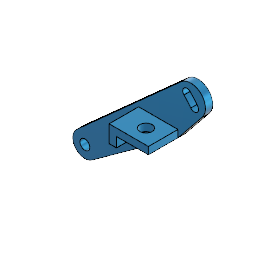
5015 Layer Fan Bracket (Autodesk Fusion 360 design; units mm, degrees)
Autodesk Fusion 360 part; units mm, degrees
ref_plane "WorkPlane1" through (0, 0, 0) normal (0, 0, 1) x (1, 0, 0)
sketch "Sketch1" plane through (0, 0, 0) normal (0, 0, 1) x (1, 0, 0)
  circle A0 centre (-26.3807, -22.7935) radius 5
  circle A1 centre (16.75, 14.4724) radius 6
  circle A2 centre (-26.3807, -22.7935) radius 2
  circle A3 centre (16.75, 14.4724) radius 1.75 construction
  line L0 (0, 0) -> (19.9948, 0) construction
  line L1 (-26.3807, -22.7935) -> (16.75, 14.4724) construction
  line L2 (22.75, 14.4724) -> (30.5, 14.4724) construction
  line L3 (-1.5, 1.4724) -> (-1.5, -1.5276)
  line L4 (11.5, -1.5276) -> (-1.5, -1.5276)
  line L5 (11.5, -1.5276) -> (11.5, 1.4724)
  line L6 (-1.5, 1.4724) -> (11.5, 1.4724)
  arc A4 (-24.5603, -21.835) -> (-27.5407, -24.5029) centre (-26.0505, -23.169) ccw construction
  arc A5 (-28.5639, -23.3119) -> (-25.4917, -20.7503) centre (-27.0278, -22.0311) ccw construction
  line L7 (-29.7155, -19.068) -> (12.7482, 18.9429)
  arc A6 (19.563, 13.7492) -> (16.4427, 17.3605) centre (-4.8153, -4.1606) ccw
  arc A7 (16.7424, 11.677) -> (19.563, 13.7492) centre (18.1527, 12.7131) ccw
  arc A8 (16.7424, 11.677) -> (13.9831, 14.8705) centre (-4.8153, -4.1606) ccw
  arc A9 (16.4427, 17.3605) -> (13.9831, 14.8705) centre (15.2129, 16.1155) ccw
  arc A10 (18.1527, 12.7131) -> (15.2129, 16.1155) centre (-4.8153, -4.1606) ccw construction
  line L8 (-1.5, 1.4724) -> (-6.7689, 1.4724) construction
  line L9 (-1.5, -1.5276) -> (-10.1203, -1.5276) construction
  line L10 (11.5, 1.4724) -> (14.108, 1.4724) construction
  line L11 (21.4103, 10.6932) -> (11.5, -1.5276)
  line L12 (-23.4475, -26.8427) -> (11.5, -1.5276)
  dimension "d5477" = 10
  dimension "d5478" = 12
  dimension "d2" = 4
  dimension "d3" = 3.5
  dimension "d4" = 16.75
  dimension "d5" = 57
  dimension "d6" = 40.828
  dimension "d27" = 2.75
  dimension "d48" = 13
  dimension "d49" = 13
  dimension "d50" = 3
  dimension "d51" = 5.25
  dimension "d54" = 2
  measures "d5477" diameter of A0
  measures "d5478" diameter of A1
  measures "d2" diameter of A2
  measures "d3" diameter of A3
  measures "d4" distance of L0.start
  measures "d5" distance of L0.start
  measures "d6" angle of L0 L1
extrude "Extrude1" add sketch "Sketch1" along normal blind 3 contours A0 | L3 L4 L5 L6 | A0 A1 L7 L11 L12 | A1
extrude "Extrude5" add sketch "Sketch1" along normal blind 15 contours L3 L4 L5 L6
hole "Hole3" at (4.5, 1.4724, 9) direction (0, -1, 0) diameter 5 depth 6 tip angle 118
sketch "Sketch6" plane through (0, 1.4724, 0) normal (0, 1, 0) x (-1, 0, 0)
  circle A0 centre (-4.5, 9) radius 2.5
  line L0 (1.5, 15) -> (-11.5, 15)
  line L1 (-11.5, 15) -> (-11.5, 3)
  line L2 (1.5, 3) -> (1.5, 15)
  line L3 (-11.5, 3) -> (1.5, 3)
  line L4 (-14.5, 18) -> (-14.5, 0)
  line L5 (-14.5, 0) -> (4.5, 0)
  line L6 (4.5, 0) -> (4.5, 18)
  line L7 (4.5, 18) -> (-14.5, 18)
  line L8 (1.5, 15) -> (4.5, 15)
  line L9 (-12.7482, 0) -> (29.7155, 0)
  line L10 (29.7155, 0) -> (29.7155, 3)
  line L11 (29.7155, 3) -> (-12.7482, 3)
  line L12 (-12.7482, 3) -> (-12.7482, 0)
  dimension "d75" = 3
  measures "d75" distance of L1
extrude "Extrude7" add sketch "Sketch6" against normal blind 7 contours L2 L6 L8 L11
named bodies: "5015 Layer Fan Buddy"
